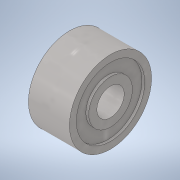
# Autodesk Inventor part: Kugellager 692-ZZ
Saved by Autodesk Inventor 2020.2 (Build 242310000, 310)
## iProperties
Part Number: Kugellager 692-ZZ
Material: Stahl, weich, geschweißt
Document SubType Name: Modeling
Designer: rYan
Mass: 0.555476 g
Surface Area: 1.35968 cm^2
Volume: 0.0707612 cm^3
Density: 7.85 g/cm^3
Appearance: Schweißnaht - Stahl - weich
Author: rYan
Autodesk Inventor part; units mm, degrees
ref_plane "YZ Plane" through (0, 0, 0) normal (1, 0, 0) x (0, 1, 0)
ref_plane "XZ Plane" through (0, 0, 0) normal (0, 1, 0) x (-1, 0, 0)
ref_plane "XY Plane" through (0, 0, 0) normal (0, 0, 1) x (1, 0, 0)
sketch "Skizze1" plane through (0, 0, 0) normal (0, 1, 0) x (-1, 0, 0)
  line L0 (1.5, 0) -> (-1.5, 0)
  line L1 (1.5, 1) -> (-1.5, 1)
  line L2 (-1.5, 1) -> (-1.5, 1.6)
  line L3 (-1.5, 1.6) -> (-1.3, 1.6)
  line L4 (-1.3, 1.6) -> (-1.3, 2.5)
  line L5 (-1.3, 2.5) -> (-1.5, 2.5)
  line L6 (-1.5, 2.5) -> (-1.5, 3)
  line L7 (-1.5, 3) -> (1.5, 3)
  line L8 (1.5, 3) -> (1.5, 2.5)
  line L9 (1.5, 2.5) -> (1.3, 2.5)
  line L10 (1.3, 2.5) -> (1.3, 1.6)
  line L11 (1.3, 1.6) -> (1.5, 1.6)
  line L12 (1.5, 1) -> (1.5, 1.6)
  line L13 (0, -0.6) -> (0, 3.6) projected
  point P0 (0, 0)
  dimension "d0" = 2
  dimension "d1" = 6
  dimension "d2" = 3
  dimension "d3" = 0.2
  dimension "d4" = 0.6
  dimension "d5" = 0.5
  constraints: 26 end point, 9 point on line, 7 perpendicular, 2 horizontal, 1 midpoint, 1 vertical, 4 other
  measures "d0" diameter of L1 L0
  measures "d1" diameter of L7 L0
  measures "d2" distance of L6.end L7.end
  measures "d3" distance of L4.end L5.end
  measures "d4" distance of L1.end L2.end
  measures "d5" distance of L5.end L6.end
revolve "Umdrehung1" add sketch "Skizze1" angle 360 about axis through (-1.5, 0, 0) along (1, 0, 0)
equation "\"d4\" = 0.1 * d1"
